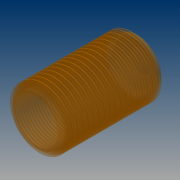
# Autodesk Inventor part: engine block
Saved by Autodesk Inventor 2014 (Build 180170000, 170)
## iProperties
Created: 2021-03-23
Part Number: engine block
Material: Lead
Document SubType Name: Modeling
Designer: Diptanshu Das
Density: 11.37 g/cm^3
Appearance: Clear - Light(3)
Author: Diptanshu Das
Autodesk Inventor part; units mm, degrees
ref_plane "YZ Plane" through (0, 0, 0) normal (1, 0, 0) x (0, 1, 0)
ref_plane "XZ Plane" through (0, 0, 0) normal (0, 1, 0) x (-1, 0, 0)
ref_plane "XY Plane" through (0, 0, 0) normal (0, 0, 1) x (1, 0, 0)
sketch "Sketch1" plane through (0, 0, 0) normal (0, 0, 1) x (1, 0, 0)
  line L0 (40, 0) -> (40, 150)
  line L1 (40, 150) -> (20, 160)
  line L2 (20, 160) -> (0, 160)
  line L3 (0, 165) -> (21.1803, 165)
  line L4 (21.1803, 165) -> (45, 153.0902)
  line L5 (45, 153.0902) -> (45, -35)
  line L6 (45, -35) -> (40, -35)
  line L7 (0, -5) -> (0, 129.0368) construction
  line L8 (45, 143.0902) -> (55, 143.0902)
  line L9 (55, 143.0902) -> (55, 141.0902)
  line L10 (55, 141.0902) -> (45, 141.0902)
  line L11 (45, 141.0902) -> (45, 143.0902)
  line L12 (45, 138.0902) -> (55, 138.0902)
  line L13 (55, 138.0902) -> (55, 136.0902)
  line L14 (55, 136.0902) -> (45, 136.0902)
  line L15 (45, 136.0902) -> (45, 138.0902)
  line L16 (45, 133.0902) -> (55, 133.0902)
  line L17 (55, 133.0902) -> (55, 131.0902)
  line L18 (55, 131.0902) -> (45, 131.0902)
  line L19 (45, 131.0902) -> (45, 133.0902)
  line L20 (45, 128.0902) -> (55, 128.0902)
  line L21 (55, 128.0902) -> (55, 126.0902)
  line L22 (55, 126.0902) -> (45, 126.0902)
  line L23 (45, 126.0902) -> (45, 128.0902)
  line L24 (45, 123.0902) -> (55, 123.0902)
  line L25 (55, 123.0902) -> (55, 121.0902)
  line L26 (55, 121.0902) -> (45, 121.0902)
  line L27 (45, 121.0902) -> (45, 123.0902)
  line L28 (45, 118.0902) -> (55, 118.0902)
  line L29 (55, 118.0902) -> (55, 116.0902)
  line L30 (55, 116.0902) -> (45, 116.0902)
  line L31 (45, 116.0902) -> (45, 118.0902)
  line L32 (45, 113.0902) -> (55, 113.0902)
  line L33 (55, 113.0902) -> (55, 111.0902)
  line L34 (55, 111.0902) -> (45, 111.0902)
  line L35 (45, 111.0902) -> (45, 113.0902)
  line L36 (45, 108.0902) -> (55, 108.0902)
  line L37 (55, 108.0902) -> (55, 106.0902)
  line L38 (55, 106.0902) -> (45, 106.0902)
  line L39 (45, 106.0902) -> (45, 108.0902)
  line L40 (45, 103.0902) -> (55, 103.0902)
  line L41 (55, 103.0902) -> (55, 101.0902)
  line L42 (55, 101.0902) -> (45, 101.0902)
  line L43 (45, 101.0902) -> (45, 103.0902)
  line L44 (45, 98.0902) -> (55, 98.0902)
  line L45 (55, 98.0902) -> (55, 96.0902)
  line L46 (55, 96.0902) -> (45, 96.0902)
  line L47 (45, 96.0902) -> (45, 98.0902)
  line L48 (0, 160) -> (0, 165)
  line L49 (45, 91.0902) -> (45, 93.0902)
  line L50 (55, 91.0902) -> (45, 91.0902)
  line L51 (45, 93.0902) -> (55, 93.0902)
  line L52 (55, 93.0902) -> (55, 91.0902)
  line L53 (45, 86.0902) -> (45, 88.0902)
  line L54 (55, 86.0902) -> (45, 86.0902)
  line L55 (45, 88.0902) -> (55, 88.0902)
  line L56 (55, 88.0902) -> (55, 86.0902)
  line L57 (45, 81.0902) -> (45, 83.0902)
  line L58 (55, 81.0902) -> (45, 81.0902)
  line L59 (45, 83.0902) -> (55, 83.0902)
  line L60 (55, 83.0902) -> (55, 81.0902)
  line L61 (45, 76.0902) -> (45, 78.0902)
  line L62 (55, 76.0902) -> (45, 76.0902)
  line L63 (45, 78.0902) -> (55, 78.0902)
  line L64 (55, 78.0902) -> (55, 76.0902)
  line L65 (45, 71.0902) -> (45, 73.0902)
  line L66 (55, 71.0902) -> (45, 71.0902)
  line L67 (45, 73.0902) -> (55, 73.0902)
  line L68 (55, 73.0902) -> (55, 71.0902)
  line L69 (45, 66.0902) -> (45, 68.0902)
  line L70 (55, 66.0902) -> (45, 66.0902)
  line L71 (45, 68.0902) -> (55, 68.0902)
  line L72 (55, 68.0902) -> (55, 66.0902)
  line L73 (45, 61.0902) -> (45, 63.0902)
  line L74 (55, 61.0902) -> (45, 61.0902)
  line L75 (45, 63.0902) -> (55, 63.0902)
  line L76 (55, 63.0902) -> (55, 61.0902)
  line L77 (45, 56.0902) -> (45, 58.0902)
  line L78 (55, 56.0902) -> (45, 56.0902)
  line L79 (45, 58.0902) -> (55, 58.0902)
  line L80 (55, 58.0902) -> (55, 56.0902)
  line L81 (40, 0) -> (40, -35)
  line L82 (45, 51.0902) -> (45, 53.0902)
  line L83 (45, 53.0902) -> (55, 53.0902)
  line L84 (55, 51.0902) -> (45, 51.0902)
  line L85 (55, 53.0902) -> (55, 51.0902)
  line L86 (45, 46.0902) -> (45, 48.0902)
  line L87 (45, 48.0902) -> (55, 48.0902)
  line L88 (55, 46.0902) -> (45, 46.0902)
  line L89 (55, 48.0902) -> (55, 46.0902)
  line L90 (45, 41.0902) -> (45, 43.0902)
  line L91 (45, 43.0902) -> (55, 43.0902)
  line L92 (55, 41.0902) -> (45, 41.0902)
  line L93 (55, 43.0902) -> (55, 41.0902)
  line L94 (45, 36.0902) -> (45, 38.0902)
  line L95 (45, 38.0902) -> (55, 38.0902)
  line L96 (55, 36.0902) -> (45, 36.0902)
  line L97 (55, 38.0902) -> (55, 36.0902)
  line L98 (45, 31.0902) -> (45, 33.0902)
  line L99 (45, 33.0902) -> (55, 33.0902)
  line L100 (55, 31.0902) -> (45, 31.0902)
  line L101 (55, 33.0902) -> (55, 31.0902)
  line L102 (45, 26.0902) -> (45, 28.0902)
  line L103 (45, 28.0902) -> (55, 28.0902)
  line L104 (55, 26.0902) -> (45, 26.0902)
  line L105 (55, 28.0902) -> (55, 26.0902)
  line L106 (45, 21.0902) -> (45, 23.0902)
  line L107 (45, 23.0902) -> (55, 23.0902)
  line L108 (55, 21.0902) -> (45, 21.0902)
  line L109 (55, 23.0902) -> (55, 21.0902)
  line L110 (45, 16.0902) -> (45, 18.0902)
  line L111 (45, 18.0902) -> (55, 18.0902)
  line L112 (55, 16.0902) -> (45, 16.0902)
  line L113 (55, 18.0902) -> (55, 16.0902)
  line L114 (45, 11.0902) -> (45, 13.0902)
  line L115 (45, 13.0902) -> (55, 13.0902)
  line L116 (55, 11.0902) -> (45, 11.0902)
  line L117 (55, 13.0902) -> (55, 11.0902)
  line L118 (55, 8.0902) -> (55, 6.0902)
  line L119 (45, 8.0902) -> (55, 8.0902)
  line L120 (55, 6.0902) -> (45, 6.0902)
  line L121 (45, 6.0902) -> (45, 8.0902)
  line L122 (55, 3.0902) -> (55, 1.0902)
  line L123 (45, 3.0902) -> (55, 3.0902)
  line L124 (55, 1.0902) -> (45, 1.0902)
  line L125 (45, 1.0902) -> (45, 3.0902)
  line L126 (55, -1.9098) -> (55, -3.9098)
  line L127 (45, -1.9098) -> (55, -1.9098)
  line L128 (55, -3.9098) -> (45, -3.9098)
  line L129 (45, -3.9098) -> (45, -1.9098)
  line L130 (45, -8.9098) -> (45, -6.9098)
  line L131 (45, -6.9098) -> (55, -6.9098)
  line L132 (55, -6.9098) -> (55, -8.9098)
  line L133 (55, -8.9098) -> (45, -8.9098)
  line L134 (45, -13.9098) -> (45, -11.9098)
  line L135 (45, -11.9098) -> (55, -11.9098)
  line L136 (55, -11.9098) -> (55, -13.9098)
  line L137 (55, -13.9098) -> (45, -13.9098)
  line L138 (45, -18.9098) -> (45, -16.9098)
  line L139 (45, -16.9098) -> (55, -16.9098)
  line L140 (55, -16.9098) -> (55, -18.9098)
  line L141 (55, -18.9098) -> (45, -18.9098)
  line L142 (45, -23.9098) -> (45, -21.9098)
  line L143 (45, -21.9098) -> (55, -21.9098)
  line L144 (55, -21.9098) -> (55, -23.9098)
  line L145 (55, -23.9098) -> (45, -23.9098)
  line L146 (45, -28.9098) -> (45, -26.9098)
  line L147 (45, -26.9098) -> (55, -26.9098)
  line L148 (55, -26.9098) -> (55, -28.9098)
  line L149 (55, -28.9098) -> (45, -28.9098)
  point P0 (0, 0)
  dimension "d34" = 40
  dimension "d36" = 20
  dimension "d37" = 10
  dimension "d38" = 5
  dimension "d39" = 10
  dimension "d40" = 2
  dimension "d41" = 10
  dimension "d42" = 10
  dimension "d43" = 2
  dimension "d44" = 10
  dimension "d45" = 2
  dimension "d46" = 10
  dimension "d47" = 2
  dimension "d48" = 10
  dimension "d49" = 2
  dimension "d50" = 10
  dimension "d51" = 2
  dimension "d52" = 10
  dimension "d53" = 2
  dimension "d54" = 10
  dimension "d55" = 2
  dimension "d56" = 10
  dimension "d57" = 2
  dimension "d59" = 2
  dimension "d62" = 3
  dimension "d63" = 3
  dimension "d64" = 3
  dimension "d65" = 3
  dimension "d66" = 3
  dimension "d67" = 3
  dimension "d68" = 3
  dimension "d69" = 3
  dimension "d70" = 3
  dimension "d73" = 2
  dimension "d74" = 2
  dimension "d75" = 2
  dimension "d76" = 2
  dimension "d77" = 2
  dimension "d78" = 2
  dimension "d79" = 2
  dimension "d80" = 2
  dimension "d81" = 3
  dimension "d82" = 10
  dimension "d83" = 3
  dimension "d84" = 3
  dimension "d85" = 3
  dimension "d86" = 3
  dimension "d87" = 3
  dimension "d88" = 3
  dimension "d89" = 3
  dimension "d90" = 195
  dimension "d91" = 2
  dimension "d92" = 2
  dimension "d93" = 2
  dimension "d94" = 2
  dimension "d95" = 2
  dimension "d96" = 2
  dimension "d97" = 2
  dimension "d98" = 2
  dimension "d99" = 2
  dimension "d101" = 3
  dimension "d102" = 3
  dimension "d103" = 3
  dimension "d104" = 3
  constraints: 300 end point, 71 parallel, 38 perpendicular, 35 collinear, 35 horizontal, 4 point on line, 2 other
  measures "d34" distance of point (0, 0) L0.start
  measures "d36" distance of L1.end L2.end
  measures "d37" vertical distance of L0.end L1.end
  measures "d38" distance between parallel lines of L0 L5
  measures "d39" distance of L9.end L10.end
  measures "d40" distance of L8.end L9.end
  measures "d41" distance from line of L8 L4.end
  measures "d42" distance of L14.start L15.start
  measures "d43" distance of L12.end L14.start
  measures "d44" distance of L18.start L19.start
  measures "d45" distance of L16.end L18.start
  measures "d46" distance of L22.start L23.start
  measures "d47" distance of L20.end L22.start
  measures "d48" distance of L26.start L27.start
  measures "d49" distance of L24.end L26.start
  measures "d50" distance of L30.start L31.start
  measures "d51" distance of L28.end L30.start
  measures "d52" distance of L34.start L35.start
  measures "d53" distance of L32.end L34.start
  measures "d54" distance of L38.start L39.start
  measures "d55" distance of L36.end L38.start
  measures "d56" distance of L42.start L43.start
  measures "d57" distance of L40.end L42.start
  measures "d59" distance of L44.end L46.start
  measures "d62" distance between parallel lines of L10 L12
  measures "d63" distance between parallel lines of L16 L14
  measures "d64" distance between parallel lines of L18 L20
  measures "d65" distance between parallel lines of L22 L24
  measures "d66" distance between parallel lines of L26 L28
  measures "d67" distance between parallel lines of L30 L32
  measures "d68" distance between parallel lines of L34 L36
  measures "d69" distance between parallel lines of L38 L40
  measures "d70" distance between parallel lines of L42 L44
  measures "d73" distance of L51.end L50.start
  measures "d74" distance of L55.end L54.start
  measures "d75" distance of L59.end L58.start
  measures "d76" distance of L63.end L62.start
  measures "d77" distance of L67.end L66.start
  measures "d78" distance of L71.end L70.start
  measures "d79" distance of L75.end L74.start
  measures "d80" distance of L79.end L78.start
  measures "d81" distance between parallel lines of L51 L46
  measures "d82" distance of L50.start L49.start
  measures "d83" distance between parallel lines of L55 L50
  measures "d84" distance between parallel lines of L59 L54
  measures "d85" distance between parallel lines of L63 L58
  measures "d86" distance between parallel lines of L67 L62
  measures "d87" distance between parallel lines of L71 L66
  measures "d88" distance between parallel lines of L70 L75
  measures "d89" distance between parallel lines of L79 L74
  measures "d90" distance from line of L6.end L2
  measures "d91" distance of L85.start L85.end
  measures "d92" distance of L89.start L89.end
  measures "d93" distance of L93.start L93.end
  measures "d94" distance of L97.start L97.end
  measures "d95" distance of L101.start L101.end
  measures "d96" distance of L105.start L105.end
  measures "d97" distance of L109.start L109.end
  measures "d98" distance of L113.start L113.end
  measures "d99" distance of L117.start L117.end
  measures "d101" distance between parallel lines of L83 L78
  measures "d102" distance between parallel lines of L87 L84
  measures "d103" distance between parallel lines of L91 L88
  measures "d104" distance between parallel lines of L95 L92
revolve "Revolution1" add sketch "Sketch1" angle 360 about axis through (0, -5, 0) along (0, 1, 0)
body "Solid1"
